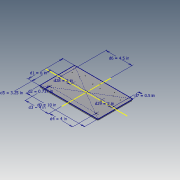
# Autodesk Inventor part: Standard
Saved by Autodesk Inventor 2020.3 (Build 243373000, 373)
## iProperties
RuleStatus: InUse
AfterDocSave0: file://Part Number Cleaner
Created: 2023-01-23
Material: Generic
Catalog Web Link: https://www.janelia.org/
Vendor: HHMI: JRC - jET
Document SubType Name: Modeling
Designer: arnoldj
Density: 1 g/cm^3
Appearance: Default
DESIGN DEPARTMENT: HHMI: JRC - jET
ALTERED ITEM PART NUMBER: N/A
ALTERED ITEM VENDOR: N/A
ALTERED ITEM DESCRIPTION: N/A
Title: Standard
Author: arnoldj
Revision Number: 0
Autodesk Inventor part; units mm, degrees
ref_plane "YZ Plane" through (0, 0, 0) normal (1, 0, 0) x (0, 1, 0)
ref_plane "XZ Plane" through (0, 0, 0) normal (0, 1, 0) x (-1, 0, 0)
ref_plane "XY Plane" through (0, 0, 0) normal (0, 0, 1) x (1, 0, 0)
sketch "Sketch1" plane through (0, 0, 0) normal (0, 1, 0) x (-1, 0, 0)
  line L0 (0, -106.68) -> (0, 106.68) projected
  line L1 (-177.8, 0) -> (177.8, 0) projected
  line L2 (-127, -76.2) -> (127, -76.2)
  line L3 (127, -76.2) -> (127, 76.2)
  line L4 (127, 76.2) -> (-127, 76.2)
  line L5 (-127, 76.2) -> (-127, -76.2)
  line L6 (-127, -76.2) -> (127, 76.2) construction
  line L7 (127, -76.2) -> (-127, 76.2) construction
  line L8 (101.6, 57.4802) -> (-101.6, 57.4802) construction
  line L9 (114.3, -6.35) -> (-114.3, -6.35) construction
  point P0 (0, 0)
  point P1 (0, -6.35)
  point P2 (63.5, -6.35)
  point P3 (-63.5, -6.35)
  dimension "d0" = 254
  dimension "d1" = 152.4
  dimension "d2" = 18.7198
  dimension "d3" = 101.6
  dimension "d4" = 101.6
  dimension "d5" = 82.55
  dimension "d6" = 114.3
  dimension "d7" = 12.7
  dimension "d28" = 50.8
  dimension "d29" = 50.8
  constraints: 16 end point, 3 coincident, 3 horizontal, 3 midpoint, 2 parallel, 2 point on line, 1 perpendicular
  measures "d0" distance of L3.end L4.end
  measures "d1" distance of L2.end L3.end
  measures "d2" distance from line of L8.start L4
  measures "d3" distance from line of L0 L8.start
  measures "d4" distance from line of L0 point (-101.6, 57.48)
  measures "d5" distance between parallel lines of L4 L9
  measures "d6" distance from line of L0 point (114.3, -6.35)
  measures "d7" distance from line of point (-114.3, -6.35) L5
  measures "d28" distance of L9.start point (63.5, -6.35)
  measures "d29" distance of point (-63.5, -6.35) L9.end
extrude "Extrusion1" add sketch "Sketch1" against normal blind 5.842
hole "Hole1" at (-101.6, 0, 57.4802) at (101.6, 0, 57.4802) direction (0, -1, 0) diameter 6.477 end through all
hole "Hole2" at (-114.3, 0, -6.35) at (114.3, 0, -6.35) at (0, 0, -6.35) at (63.5, 0, -6.35) at (-63.5, 0, -6.35) direction (0, -1, 0) diameter 3.1242 end through all
pattern_linear "Rectangular Pattern1" count 2 spacing 53.975 along (0, 0, -1) of "Hole2"
sketch "Sketch2" plane through (0, 0, 0) normal (0, 1, 0) x (1, 0, 0)
  circle A0 centre (-114.3, 60.325) radius 1.5621 projected
  circle A1 centre (-63.5, 60.325) radius 1.5621 projected
  line L0 (-114.3, 60.325) -> (-63.5, 60.325) construction
  line L1 (-88.9, 60.325) -> (-88.9, 44.45) construction
  line L2 (-104.775, 45.0718) -> (-73.025, 45.0718) construction
  point P0 (0, 0)
  dimension "d31" = 31.75
  dimension "d32" = 15.875
  dimension "d33" = 15.875
  constraints: 6 end point, 2 coincident, 2 horizontal, 1 midpoint, 1 vertical
  measures "d31" distance of L2.start L2.end
  measures "d32" distance from line of L1 L2.start
  measures "d33" distance of L1.start L1.end
hole "Hole3" at (-104.775, 0, -45.0718) at (-73.025, 0, -45.0718) direction (0, -1, 0) diameter 3.1242 end through all
fillet "Fillet1" radius 6.35 4 edges at (127, -2.921, 76.2) (127, -2.921, -76.2) (-127, -2.921, 76.2) (-127, -2.921, -76.2)
pattern_linear "Rectangular Pattern2" count 3 spacing 88.9 along (1, 0, 0) of "Hole3"
equation "\"d32\" = 0.5 * d31"
body "Solid1"
